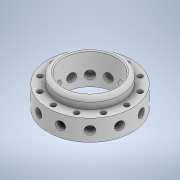
# Autodesk Inventor part: diaphragm
Saved by Autodesk Inventor 2021 (Build 250183000, 183)
## iProperties
Created: 2022-10-28
Part Number: diaphragm
Material: Generic
Document SubType Name: Modeling
Designer: warre
Density: 1 g/cm^3
Appearance: Default
Author: warre
Autodesk Inventor part; units mm, degrees
ref_plane "YZ Plane" through (0, 0, 0) normal (1, 0, 0) x (0, 1, 0)
ref_plane "XZ Plane" through (0, 0, 0) normal (0, 1, 0) x (-1, 0, 0)
sketch "Sketch1" plane through (0, 0, 0) normal (0, 1, 0) x (-1, 0, 0)
  circle A0 centre (0, 0) radius 25
  circle A1 centre (0, 0) radius 40
  dimension "d0" = 50
  dimension "d1" = 80
  constraints: 2 centre point, 2 coincident
  measures "d0" diameter of A0
  measures "d1" diameter of A1
extrude "Extrusion1" add sketch "Sketch1" along normal blind 20
sketch "Sketch2" plane through (0, 20, 0) normal (0, 1, 0) x (1, 0, 0)
  circle A0 centre (0, 0) radius 25
  circle A1 centre (0, 0) radius 30
  dimension "d4" = 60
  constraints: 2 centre point, 2 coincident
  measures "d4" diameter of A1
extrude "Extrusion2" add sketch "Sketch2" along normal blind 10
fillet "Fillet1" radius 4 1 edges at (-30, 30, 0)
fillet "Fillet1" radius 1 1 edges at (-25, 30, 0)
sketch "Sketch3" plane through (0, 20, 0) normal (0, 1, 0) x (1, 0, 0)
  circle A0 centre (0, 0) radius 30 construction
  line L0 (0, 30) -> (0, 35) construction
  circle A1 centre (0, 0) radius 35
  circle A2 centre (0, 35) radius 2.4
  circle A3 centre (-17.5, 30.3109) radius 2.4
  circle A4 centre (-30.3109, 17.5) radius 2.4
  circle A5 centre (-35, 0) radius 2.4
  circle A6 centre (-30.3109, -17.5) radius 2.4
  circle A7 centre (-17.5, -30.3109) radius 2.4
  circle A8 centre (0, -35) radius 2.4
  circle A9 centre (17.5, -30.3109) radius 2.4
  circle A10 centre (30.3109, -17.5) radius 2.4
  circle A11 centre (35, 0) radius 2.4
  circle A12 centre (30.3109, 17.5) radius 2.4
  circle A13 centre (17.5, 30.3109) radius 2.4
  line L1 (-35, 0) -> (-40, 0) construction
  circle A14 centre (0, 0) radius 40 construction
  dimension "d8" = 5
  dimension "d9" = 4.8
  dimension "d12" = 360
  constraints: 12 centre point, 4 end point, 2 coincident, 2 vertical alignment, 1 horizontal, 1 horizontal alignment, 1 vertical, 29 other
  measures "d8" distance of L0.start L0.end
  measures "d9" diameter of A2
extrude "Extrusion3" cut sketch "Sketch3" against normal blind 15 contours A1 A11 | A1 A11 | A12 A1 | A1 A12 | A10 A1 | A1 A10 | A13 A1 | A1 A13 | A9 A1 | A1 A9 | A2 A1 | A1 A2 | A8 A1 | A1 A8 | A3 A1 | A1 A3 | A7 A1 | A1 A7 | A4 A1 | A1 A4 | A6 A1 | A1 A6 | A5 A1 | A1 A5
ref_plane "Work Plane1" through (0, -10, 0) normal (0, -1, 0) x (1, 0, 0)
ref_plane "Work Plane2" through (0, 0, 40) normal (0, 0, 1) x (1, 0, 0)
sketch "Sketch6" plane through (0, 0, 40) normal (0, 0, 1) x (1, 0, 0)
  point P0 (0, 0)
pattern_of_nothing "Circular Pattern1"
sketch "Sketch7" plane through (-10.3528, 0, 38.637) normal (-0.258819, 0, 0.9659258) x (0.9659258, 0, 0.258819)
  line L0 (40, 20) -> (-40, 20) projected
  line L1 (40, 0) -> (-40, 0) projected
  line L2 (0, 20) -> (0, 0) construction
  circle A0 centre (0, 10) radius 4
  dimension "d39" = 20
  dimension "d40" = 8
  constraints: 2 end point, 2 midpoint, 1 centre point, 1 vertical
  measures "d39" distance of L2.start L2.end
  measures "d40" diameter of A0
extrude "Extrusion6" cut sketch "Sketch7" against normal through all
pattern_circular "Circular Pattern2" count 12 over 360 about axis through (0, 0, 0) along (0, 1, 0) of "Extrusion6"
sketch "Sketch8" plane through (0, 0, 0) normal (0, -1, 0) x (1, 0, 0)
  circle A0 centre (0, 35) radius 2.4 projected
  circle A1 centre (0, 35) radius 2.4 projected
  circle A2 centre (0, 35) radius 2
  circle A3 centre (-30.3109, 17.5) radius 2
  circle A4 centre (-30.3109, -17.5) radius 2
  circle A5 centre (0, -35) radius 2
  circle A6 centre (30.3109, -17.5) radius 2
  circle A7 centre (30.3109, 17.5) radius 2
  point P0 (0, 0)
  dimension "d46" = 4
  dimension "d49" = 360
  constraints: 6 centre point, 1 coincident, 13 other
  measures "d46" diameter of A2
extrude "Extrusion7" cut sketch "Sketch8" against normal blind 5 contours A2 | A3 | A4 | A5 | A6 | A7
ref_plane "Work Plane3" through (10.3528, 0, 38.637) normal (0.258819, 0, 0.9659258) x (0.9659258, 0, -0.258819)
ref_plane "Work Plane4" through (20, 0, 34.641) normal (0.5, 0, 0.8660254) x (0.8660254, 0, -0.5)
ref_plane "Work Plane5" through (28.2843, 0, 28.2843) normal (0.7071068, 0, 0.7071068) x (0.7071068, 0, -0.7071068)
ref_plane "Work Plane6" through (34.641, 0, 20) normal (0.8660254, 0, 0.5) x (0.5, 0, -0.8660254)
ref_plane "Work Plane7" through (38.637, 0, 10.3528) normal (0.9659258, 0, 0.258819) x (0.258819, 0, -0.9659258)
ref_plane "Work Plane8" through (40, 0, 0) normal (1, 0, 0) x (0, 0, -1)
ref_plane "Work Plane9" through (38.637, 0, -10.3528) normal (0.9659258, 0, -0.258819) x (-0.258819, 0, -0.9659258)
ref_plane "Work Plane10" through (34.641, 0, -20) normal (0.8660254, 0, -0.5) x (-0.5, 0, -0.8660254)
ref_plane "Work Plane11" through (28.2843, 0, -28.2843) normal (0.7071068, 0, -0.7071068) x (-0.7071068, 0, -0.7071068)
ref_plane "Work Plane12" through (20, 0, -34.641) normal (0.5, 0, -0.8660254) x (-0.8660254, 0, -0.5)
ref_plane "Work Plane13" through (10.3528, 0, -38.637) normal (0.258819, 0, -0.9659258) x (-0.9659258, 0, -0.258819)
ref_plane "Work Plane14" through (0, 0, -40) normal (0, 0, -1) x (-1, 0, 0)
ref_plane "Work Plane15" through (-10.3528, 0, -38.637) normal (-0.258819, 0, -0.9659258) x (-0.9659258, 0, 0.258819)
ref_plane "Work Plane16" through (-20, 0, -34.641) normal (-0.5, 0, -0.8660254) x (-0.8660254, 0, 0.5)
ref_plane "Work Plane17" through (-28.2843, 0, -28.2843) normal (-0.7071068, 0, -0.7071068) x (-0.7071068, 0, 0.7071068)
ref_plane "Work Plane18" through (-34.641, 0, -20) normal (-0.8660254, 0, -0.5) x (-0.5, 0, 0.8660254)
ref_plane "Work Plane19" through (-38.637, 0, -10.3528) normal (-0.9659258, 0, -0.258819) x (-0.258819, 0, 0.9659258)
ref_plane "Work Plane20" through (-40, 0, 0) normal (-1, 0, 0) x (0, 0, 1)
ref_plane "Work Plane21" through (-38.637, 0, 10.3528) normal (-0.9659258, 0, 0.258819) x (0.258819, 0, 0.9659258)
ref_plane "Work Plane22" through (-34.641, 0, 20) normal (-0.8660254, 0, 0.5) x (0.5, 0, 0.8660254)
ref_plane "Work Plane23" through (-28.2843, 0, 28.2843) normal (-0.7071068, 0, 0.7071068) x (0.7071068, 0, 0.7071068)
ref_plane "Work Plane24" through (-20, 0, 34.641) normal (-0.5, 0, 0.8660254) x (0.8660254, 0, 0.5)
ref_plane "Work Plane25" through (-10.3528, 0, 38.637) normal (-0.258819, 0, 0.9659258) x (0.9659258, 0, 0.258819)
body "Solid1"
